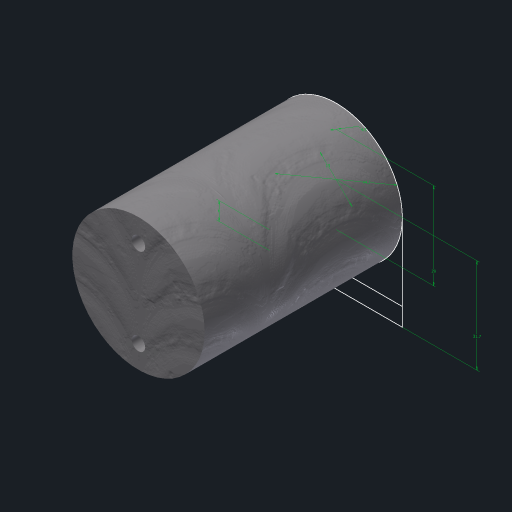
# Autodesk Inventor part: MOTOR_NUEVO_DC
Saved by Autodesk Inventor 2024.3 (Build 283343000, 343)
## iProperties
Created: 2024-08-10
Part Number: MOTOR_NUEVO_DC
Material: Steel, Mild, Welded
Document SubType Name: Modeling
Designer: Niler
Density: 7.85 g/cm^3
Appearance: Weld - Steel Mild
Author: Niler
Autodesk Inventor part; units mm, degrees
ref_plane "YZ Plane" through (0, 0, 0) normal (1, 0, 0) x (0, 1, 0)
ref_plane "XZ Plane" through (0, 0, 0) normal (0, 1, 0) x (-1, 0, 0)
ref_plane "XY Plane" through (0, 0, 0) normal (0, 0, 1) x (1, 0, 0)
sketch "Sketch1" plane through (0, 0, 0) normal (0, 0, 1) x (1, 0, 0)
  circle A0 centre (0, 0) radius 22.1
  circle A1 centre (0, 14.5) radius 2.25
  circle A2 centre (0, -14.5) radius 2.25
  line L0 (0, 14.5) -> (0, -14.5)
  circle A3 centre (0, 0) radius 7.5
  line L1 (-22.1, 0) -> (-22.1, -31.7)
  line L2 (-22.1, -31.7) -> (22.1, -31.7)
  line L3 (22.1, -31.7) -> (22.1, 0)
  line L4 (-22.1, -25.7) -> (22.1, -25.7)
  dimension "d0" = 44.2
  dimension "d1" = 29
  dimension "d2" = 4.5
  dimension "d3" = 15
  dimension "d4" = 31.7
  dimension "d5" = 6
  constraints: 10 end point, 4 centre point, 3 coincident, 3 perpendicular, 2 point on circle, 2 point on line, 2 vertical, 1 equal radius, 1 horizontal alignment, 1 midpoint, 1 tangent
  measures "d0" diameter of A0
  measures "d1" distance of L0.end L0.start
  measures "d2" diameter of A1
  measures "d3" diameter of A3
  measures "d4" distance from line of L2 point (0, 0)
  measures "d5" distance between parallel lines of L2 L4
extrude "Extrusion1" add sketch "Sketch1" along normal blind 66 contours A0 | A3 L0 | L0 A3
extrude "Extrusion2" add sketch "Sketch1" against normal blind 4.5 contours A3 L0 | L0 A3
body "Solid1"
